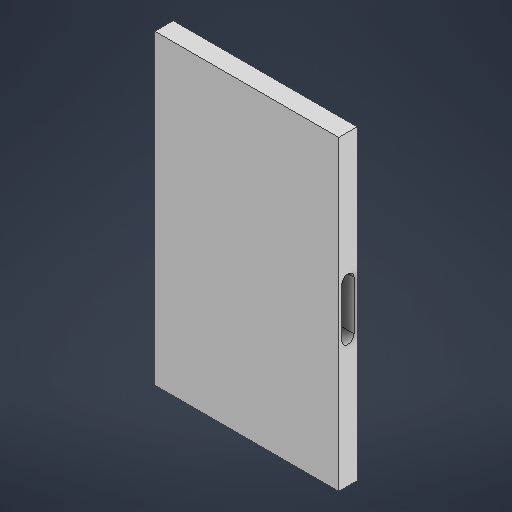
# Autodesk Inventor part: motor box 2
Saved by Autodesk Inventor 2026.2 (Build 302298010, 298A)
## iProperties
Created: 2026-04-13
Part Number: motor box 2
Material: Generic
Document SubType Name: Modeling
Designer: yasser
Density: 1 g/cm^3
Appearance: Default
Author: yasser
Autodesk Inventor part; units mm, degrees
ref_plane "YZ Plane" through (0, 0, 0) normal (1, 0, 0) x (0, 1, 0)
ref_plane "XZ Plane" through (0, 0, 0) normal (0, 1, 0) x (-1, 0, 0)
sketch "Sketch1" plane through (0, 0, 0) normal (0, 0, 1) x (1, 0, 0)
  line L0 (0, 0) -> (30, 0)
  line L1 (30, 0) -> (30, 50)
  line L2 (30, 50) -> (0, 50)
  line L3 (0, 50) -> (0, 0)
  dimension "d0" = 30
  dimension "d1" = 50
  constraints: 8 end point, 2 parallel, 1 horizontal, 1 perpendicular
  measures "d0" distance of L2.end L1.end
  measures "d1" distance of L1.end L0.end
extrude "Extrusion1" add sketch "Sketch1" along normal blind 3
sketch "Sketch2" plane through (30, 0, 0) normal (1, 0, 0) x (0, 0, -1)
  line L0 (-1.5, 30) -> (-1.5, 20) construction
  line L1 (-3, 0) -> (-3, 50) projected
  line L2 (-2.5, 29) -> (-2.5, 21)
  line L3 (-0.5, 21) -> (-0.5, 29)
  arc A0 (-0.5, 29) -> (-2.5, 29) centre (-1.5, 29) ccw
  arc A1 (-2.5, 21) -> (-0.5, 21) centre (-1.5, 21) ccw
  line L4 (0, 0) -> (0, 50) projected
  point P0 (-1.5, 25)
  point P1 (0, 25)
  dimension "d12" = 25
  dimension "d13" = 1
  dimension "d14" = 10
  dimension "d15" = 1.5
  constraints: 8 end point, 8 point on circle, 4 tangent, 2 centre point, 2 midpoint, 2 parallel, 2 point on line
  measures "d12" vertical distance of L4.start point (-1.5, 25)
  measures "d13" radius of A0
  measures "d14" distance of point (-1.5, 20) point (-1.5, 30)
  measures "d15" distance of point (0, 25) point (-1.5, 25)
extrude "Extrusion2" cut sketch "Sketch2" against normal blind 3.7
ref_plane "Work Plane1" through (15, 0, 0) normal (1, 0, 0) x (0, 0, -1)
mirror "Mirror1" about plane through (15, 0, 0) normal (1, 0, 0) of "Extrusion2"
body "Solid1"
